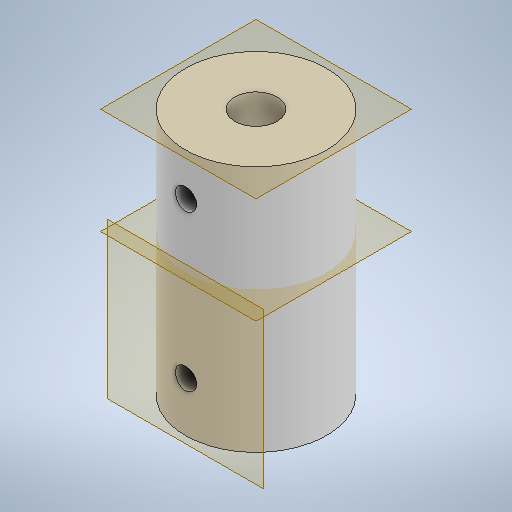
# Autodesk Inventor part: joint
Saved by Autodesk Inventor 2025.1 (Build 291241000, 241)
## iProperties
Created: 2024-11-23
Part Number: joint
Material: 一般
Document SubType Name: Modeling
Designer: dell
Density: 1 g/cm^3
Appearance: 既定
Author: dell
Autodesk Inventor part; units mm, degrees
ref_plane "YZ Plane" through (0, 0, 0) normal (1, 0, 0) x (0, 1, 0)
ref_plane "XZ Plane" through (0, 0, 0) normal (0, 1, 0) x (-1, 0, 0)
sketch "スケッチ1" plane through (0, 0, 0) normal (0, 1, 0) x (-1, 0, 0)
  circle A0 centre (0, 0) radius 10
  dimension "d0" = 20
  constraints: 1 centre point, 1 coincident
  measures "d0" diameter of A0
extrude "押し出し1" add sketch "スケッチ1" along normal blind 20
sketch "スケッチ2" plane through (0, 0, 0) normal (0, -1, 0) x (1, 0, 0)
  circle A0 centre (0, 0) radius 5.5
  dimension "d4" = 11
  constraints: 1 centre point, 1 coincident
  measures "d4" diameter of A0
hole "穴1" at (0, 0, 0) direction (0, 1, 0) diameter 11 depth 14
ref_plane "作業平面1" through (0, 0, 10) normal (0, 0, 1) x (1, 0, 0)
sketch "スケッチ3" plane through (0, 0, 10) normal (0, 0, 1) x (1, 0, 0)
  point P0 (0, 0)
  point P1 (0, 7)
hole "穴2" at (0, 7, 10) direction (0, 0, -1) diameter 3 depth 6
ref_plane "作業平面4" through (0, 20, 0) normal (0, 1, 0) x (1, 0, 0)
sketch "スケッチ5" plane through (0, 20, 0) normal (0, 1, 0) x (1, 0, 0)
  circle A0 centre (0, 0) radius 10
  constraints: 1 centre point, 1 coincident
extrude "押し出し2" add sketch "スケッチ5" along normal blind 15
ref_plane "作業平面5" through (0, 35, 0) normal (0, 1, 0) x (1, 0, 0)
sketch "スケッチ6" plane through (0, 35, 0) normal (0, 1, 0) x (1, 0, 0)
  circle A0 centre (0, 0) radius 3
  dimension "d23" = 6
  constraints: 1 centre point, 1 coincident
  measures "d23" diameter of A0
hole "穴3" at (0, 35, 0) direction (0, -1, 0) diameter 6 depth 14
sketch "スケッチ7" plane through (0, 0, 10) normal (0, 0, 1) x (1, 0, 0)
  circle A0 centre (0, 29) radius 1.5
  point P0 (0, 0)
  dimension "d31" = 3
  constraints: 1 centre point, 1 coincident
  measures "d31" diameter of A0
hole "穴4" at (0, 29, 10) direction (0, 0, -1) diameter 3 depth 8
ref_plane "作業平面7" through (0, 21, 0) normal (0, 1, 0) x (1, 0, 0)
ref_plane "作業平面8" through (0, 14, 0) normal (0, -1, 0) x (1, 0, 0)
